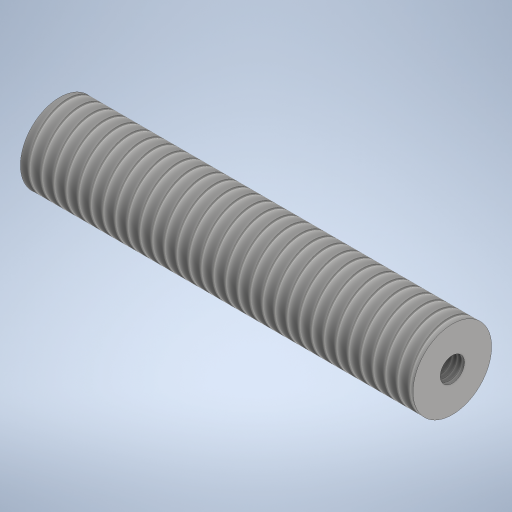
# Autodesk Inventor part: Perilla
Saved by Autodesk Inventor 2024.2 (Build 282272000, 272)
## iProperties
Created: 2025-06-19
Part Number: Perilla
Material: Genérico
Document SubType Name: Modeling
Designer: jd.castellanosq
Density: 1 g/cm^3
Appearance: Valor por defecto
Author: jd.castellanosq
Autodesk Inventor part; units mm, degrees
ref_plane "YZ Plane" through (0, 0, 0) normal (1, 0, 0) x (0, 1, 0)
ref_plane "XZ Plane" through (0, 0, 0) normal (0, 1, 0) x (-1, 0, 0)
ref_plane "XY Plane" through (0, 0, 0) normal (0, 0, 1) x (1, 0, 0)
sketch "Boceto1" plane through (0, 0, 0) normal (0, 0, 1) x (1, 0, 0)
  line L0 (-20, 0) -> (20, 0)
  line L1 (-20, 4) -> (20, 4)
  line L2 (20, 4) -> (20, 0)
  line L3 (15, 2.5) -> (20, 2.5)
  line L4 (15, 4) -> (15, 2.5)
  line L5 (-20, 4) -> (-20, 0)
  line L6 (-20, 2.5) -> (-15, 2.5)
  line L7 (-15, 2.5) -> (-15, 4)
  point P0 (0, 0)
  point P1 (0, 0)
  dimension "d0" = 8
  dimension "d13" = 5
  dimension "d22" = 5
  dimension "d30" = 20
  dimension "d31" = 40
  dimension "d38" = 5
  dimension "d39" = 5
  constraints: 16 end point, 5 point on line, 3 perpendicular, 2 coincident, 2 horizontal, 1 midpoint, 1 vertical
  measures "d0" diameter of L1 L0
  measures "d13" diameter of L3 L0
  measures "d22" distance between parallel lines of L2 L4
  measures "d30" distance from line of L5 point (0, 0)
  measures "d31" distance between parallel lines of L2 L5
  measures "d38" diameter of L6 L0
  measures "d39" distance between parallel lines of L5 L7
revolve "Revolución1" add sketch "Boceto1" angle 360 about axis through (-20, 0, 0) along (1, 0, 0)
thread "Rosca1" size "M8x1.25" class "6g" standard "ANSI Metric M Profile" full length
sketch "Boceto2" plane through (20, 0, 0) normal (1, 0, 0) x (0, 0, -1)
  point P0 (0, 0)
  point P1 (0, 0)
  constraints: 1 coincident
hole "Agujero1" at (20, 0, 0) direction (-1, 0, 0) diameter 2.459 depth 10 tip angle 118 thread size "M3x0.5" class "6H" standard "ISO Metric profile"
equation "\"d30\" = 0.5 * d31"
